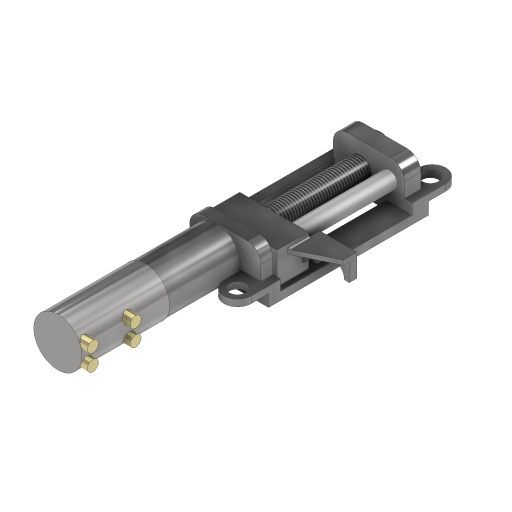
# Autodesk Inventor part: motor_lowest
Saved by Autodesk Inventor 2023 (Build 270158030, 158C)
## iProperties
Created: 2021-04-15
Part Number: motor_lowest
Material: Generic
Document SubType Name: Modeling
Designer: Robert Cobden
Density: 1 g/cm^3
Appearance: Steel Galvanized
Author: Robert Cobden
Autodesk Inventor part; units mm, degrees
sketch "Sketch1" plane through (0, 0, 0) normal (0, 1, 0) x (-1, 0, 0)
  line L0 (3.2, -7.5) -> (-4.7, -7.5)
  line L1 (-4.7, -7.5) -> (-4.7, 7.1)
  line L2 (-4.7, 7.1) -> (3.2, 7.1)
  line L3 (3.2, 7.1) -> (3.2, -7.5)
  line L4 (-2.35, 6) -> (2.35, 6)
  line L5 (2.35, 6) -> (2.35, -6)
  line L6 (2.35, -6) -> (-2.35, -6)
  line L7 (-2.35, -6) -> (-2.35, 6)
  line L8 (-2.35, 6) -> (2.35, -6) construction
  line L9 (2.35, 6) -> (-2.35, -6) construction
  point P0 (0, 0)
  dimension "d0" = 7.9
  dimension "d1" = 14.6
  dimension "d2" = 4.7
  dimension "d3" = 12
  dimension "d4" = 0.85
  dimension "d5" = 1.5
  constraints: 20 end point, 4 parallel, 2 horizontal, 2 midpoint, 2 perpendicular
  measures "d0" distance of L1.end L2.end
  measures "d1" distance of L0.end L1.end
  measures "d2" distance of L5.end L6.end
  measures "d3" distance of L4.end L5.end
  measures "d4" distance between parallel lines of L5 L3
  measures "d5" distance between parallel lines of L0 L6
extrude "Extrusion1" add sketch "Sketch1" along normal blind 0.75
sketch "Sketch2" plane through (0, 0.75, 0) normal (0, 1, 0) x (1, 0, 0)
  line L0 (-3.2, -7.1) -> (4.7, -7.1) projected
  line L1 (4.7, -7.1) -> (4.7, 7.5) projected
  line L2 (4.7, 7.5) -> (-3.2, 7.5) projected
  line L3 (-3.2, 7.5) -> (-3.2, -7.1) projected
  line L4 (2.35, -6) -> (-2.35, -6) projected
  line L5 (-2.35, -6) -> (-2.35, 6) projected
  line L6 (-2.35, 6) -> (2.35, 6) projected
  line L7 (2.35, 6) -> (2.35, -6) projected
  line L8 (-2.35, 6) -> (2.35, 6) projected
  line L9 (2.35, 6) -> (4.7, 6)
  line L10 (4.7, -7.1) -> (4.7, 7.5) projected
  line L11 (2.35, -6) -> (-2.35, -6) projected
  line L12 (2.35, -6) -> (4.7, -6)
  point P0 (0, 0)
  constraints: 4 end point, 2 perpendicular, 2 point on line
extrude "Extrusion2" add sketch "Sketch2" along normal blind 0.95 contours L3 L2 L1 L9 L6 L5 L4 L12 L0
sketch "Sketch3" plane through (0, 1.7, 0) normal (0, 1, 0) x (1, 0, 0)
  line L0 (4.7, -7.1) -> (4.7, -6) projected
  line L1 (4.7, -6) -> (-2.35, -6) projected
  line L2 (-2.35, -6) -> (-2.35, 6) projected
  line L3 (-2.35, 6) -> (4.7, 6) projected
  line L4 (4.7, 6) -> (4.7, 7.5) projected
  line L5 (4.7, 7.5) -> (-3.2, 7.5) projected
  line L6 (-3.2, 7.5) -> (-3.2, -7.1) projected
  line L7 (-3.2, -7.1) -> (4.7, -7.1) projected
  line L8 (4.7, 6) -> (4.7, 7.5) projected
  line L9 (4.7, 7.5) -> (2.2, 7.5)
  line L10 (2.2, 7.5) -> (2.2, 10.34)
  line L11 (2.2, 10.34) -> (4.7, 10.34)
  line L12 (4.7, 10.34) -> (4.7, 7.5)
  line L13 (4.7, 7.5) -> (-3.2, 7.5) projected
  line L14 (-3.2, 7.5) -> (-1.0999, 7.5)
  line L15 (-1.0999, 7.5) -> (-1.0999, 10.2)
  line L16 (-1.0999, 10.2) -> (-3.2, 10.2)
  line L17 (-3.2, 10.2) -> (-3.2, 7.5)
  circle A0 centre (-2.3499, 8.95) radius 1.25
  circle A1 centre (-2.3499, 8.95) radius 0.75
  circle A2 centre (3.45, 8.92) radius 0.75
  line L18 (2.2, 10.34) -> (4.7, 7.5) construction
  line L19 (4.7, -7.1) -> (4.7, 7.5) projected
  line L20 (4.7, -7.1) -> (2.2, -7.1)
  line L21 (2.2, -7.1) -> (2.2, -9.93)
  line L22 (2.2, -9.93) -> (4.7, -9.93)
  line L23 (4.7, -9.93) -> (4.7, -7.1)
  circle A3 centre (3.45, -8.68) radius 0.75
  line L24 (3.45, -9.93) -> (3.45, -8.68) construction
  point P0 (0, 0)
  point P1 (2.2, 7.5)
  point P2 (-3.2, 8.0336)
  point P3 (-1.0999, 7.5)
  point P4 (-2.3499, 10.2)
  dimension "d10" = 2.5
  dimension "d11" = 2.84
  dimension "d12" = 2.1001
  dimension "d13" = 2.7
  dimension "d14" = 2.5
  dimension "d16" = 1.5
  dimension "d17" = 2.5
  dimension "d18" = 2.83
  dimension "d20" = 1.25
  dimension "d38" = 5.8
  dimension "d39" = 8.2999
  dimension "d40" = 7.3
  dimension "d41" = 19.1
  dimension "d42" = 2.17
  dimension "d43" = 2.2
  constraints: 28 end point, 6 parallel, 4 centre point, 3 horizontal, 3 perpendicular, 2 coincident, 2 equal radius, 2 midpoint, 2 tangent, 1 vertical
  measures "d10" distance of L10.end L11.end
  measures "d11" distance of L9.end L10.end
  measures "d12" distance of L16.end L15.end
  measures "d13" distance of L15.end L14.end
  measures "d14" diameter of A0
  measures "d16" diameter of A2
  measures "d17" distance of L22.end L21.end
  measures "d18" distance of L21.end L20.end
  measures "d20" distance of L24.start L24.end
  measures "d38" distance of A2.centre A0.centre
extrude "Extrusion3" add sketch "Sketch3" against normal blind 0.6 contours L23 L22 L21 L7 | L5 L10 L11 L12
extrude "Extrusion4" add sketch "Sketch3" against normal blind 0.4 contours L17 A0 L15 L5 | A0 L17 | L17 A0 | A0 L16 L15
sketch "Sketch4" plane through (0, 1.7, 0) normal (0, 1, 0) x (1, 0, 0)
  circle A0 centre (-2.3499, 8.95) radius 0.75 construction
  circle A1 centre (3.45, -8.68) radius 0.75 construction
  circle A2 centre (3.45, 8.92) radius 0.75 construction
  line L0 (4.7, -9.93) -> (4.7, -6) construction
  line L1 (4.7, -6) -> (-2.35, -6) construction
  line L2 (-2.35, -6) -> (-2.35, 6) construction
  line L3 (-2.35, 6) -> (4.7, 6) construction
  line L4 (4.7, 6) -> (4.7, 10.34) construction
  line L5 (4.7, 10.34) -> (2.2, 10.34) construction
  line L6 (2.2, 10.34) -> (2.2, 7.5) construction
  line L7 (2.2, 7.5) -> (-1.0999, 7.5) construction
  line L8 (-1.0999, 7.5) -> (-1.0999, 10.2) construction
  line L9 (-1.0999, 10.2) -> (-2.3499, 10.2) construction
  arc A3 (-2.3499, 10.2) -> (-3.2, 8.0336) centre (-2.3499, 8.95) ccw construction
  line L10 (-3.2, 8.0336) -> (-3.2, -7.1) construction
  line L11 (-3.2, -7.1) -> (2.2, -7.1) construction
  line L12 (2.2, -7.1) -> (2.2, -9.93) construction
  line L13 (2.2, -9.93) -> (4.7, -9.93) construction
  line L14 (-2.5, 7.5) -> (4, 7.5)
  line L15 (4, 7.5) -> (4, 6)
  line L16 (4, 6) -> (-2.5, 6)
  line L17 (-2.5, 6) -> (-2.5, 7.5)
  line L18 (2.2, 7.5) -> (-1.0999, 7.5) projected
  line L19 (-2.35, 6) -> (4.7, 6) projected
  line L20 (-3.2, 7.5) -> (-3.2, -7.1) construction
  line L21 (-3.2, -1.2421) -> (4.7, -1.2421) construction
  line L22 (-3.2, 8.0336) -> (-3.2, -7.1) construction
  line L23 (4.7, 6) -> (4.7, 10.34) construction
  line L24 (0.75, -1.2421) -> (0.75, 6) construction
  line L25 (-2.5, -6) -> (4, -6)
  line L26 (4, -6) -> (4, -7.1)
  line L27 (4, -7.1) -> (-2.5, -7.1)
  line L28 (-2.5, -7.1) -> (-2.5, -6)
  line L29 (0.75, -1.2421) -> (0.75, -6) construction
  line L30 (4.7, -6) -> (-2.35, -6) construction
  line L31 (-3.2, -7.1) -> (2.2, -7.1) construction
  point P0 (0, 0)
  dimension "d25" = 6.5
  dimension "d26" = 6.5
  constraints: 22 end point, 5 point on line, 4 parallel, 4 perpendicular, 3 midpoint, 2 horizontal, 1 collinear, 1 vertical
  measures "d25" distance of L14.start L14.end
  measures "d26" distance of L26.end L27.end
extrude "Extrusion5" add sketch "Sketch4" along normal blind 2.6
fillet "Fillet1" radius 1.25 5 edges at (2.2, 1.4, 9.93) (4.7, 1.4, 9.93) (4.7, 1.4, -10.34) (2.2, 1.4, -10.34) (-1.0999, 1.5, -10.2)
fillet "Fillet1" radius 1.25 4 edges at (4, 4.3, 6.55) (-2.5, 4.3, 6.55) (-2.5, 4.3, -6.75) (4, 4.3, -6.75)
sketch "Sketch5" plane through (0, 0, 0) normal (0, -1, 0) x (1, 0, 0)
  circle A0 centre (3.55, 5.25) radius 0.55
  circle A1 centre (3.55, -4.8) radius 0.55
  line L0 (4.7, 7.1) -> (4.7, -7.5) projected
  line L1 (3.55, 5.25) -> (3.55, -4.8) construction
  line L2 (4.7, -7.5) -> (-3.2, -7.5) construction
  point P0 (0, 0)
  dimension "d31" = 1.1
  dimension "d33" = 1.7
  dimension "d34" = 11.15
  dimension "d35" = 3.25
  constraints: 2 centre point, 2 end point, 1 equal radius, 1 vertical
  measures "d31" diameter of A1
extrude "Extrusion6" add sketch "Sketch5" along normal blind 0.29
sketch "Sketch6" plane through (-2.35, 0, -6) normal (0, 0, 1) x (1, 0, 0)
  circle A0 centre (4.9823, 2.55) radius 0.75
  circle A1 centre (2.32, 2.15) radius 1
  line L0 (6.35, 1.7) -> (6.35, 3.05) projected
  line L1 (0, 0) -> (4.7, 0) projected
  circle A2 centre (2.32, 2.15) radius 2.15 construction
  line L2 (7.05, 0.75) -> (7.05, 1.7) projected
  line L3 (1.1, 4.3) -> (5.1, 4.3) projected
  point P0 (2.35, 0)
  dimension "d44" = 2.1177
  dimension "d45" = 1.5
  dimension "d46" = 3.3
  dimension "d47" = 2
  dimension "d49" = 4.3
  dimension "d50" = 6.88
  constraints: 3 centre point, 1 coincident, 1 tangent
  measures "d45" diameter of A0
  measures "d47" diameter of A1
  measures "d49" diameter of A2
extrude "Extrusion7" cut sketch "Sketch6" along normal blind 13.1 and the other way blind 1.5 contours A1
extrude "Extrusion8" add sketch "Sketch6" along normal blind 12 contours A0
extrude "Extrusion9" add sketch "Sketch6" along normal blind 13.1 and the other way blind 1.5 separate body contours A1
thread "Thread1" size "M2x0.25" class "6g" standard "ANSI Metric M Profile" full length
sketch "Sketch9" plane through (-3.2, 0, 7.1) normal (0, 0, 1) x (1, 0, 0)
  circle A0 centre (3.17, 2.15) radius 1 construction
  circle A1 centre (3.17, 2.15) radius 2.15
  line L0 (1.95, 4.3) -> (5.95, 4.3) projected
  point P0 (3.2, 0)
  constraints: 1 centre point, 1 coincident, 1 tangent
extrude "Extrusion13" add sketch "Sketch9" along normal blind 6.5 separate body
sketch "Sketch7" plane through (-3.2, 0, 13.6) normal (0, 0, 1) x (1, 0, 0)
  circle A0 centre (3.17, 2.15) radius 1 construction
  circle A1 centre (3.17, 2.15) radius 2.2
  point P0 (3.2, 0)
  dimension "d76" = 4.4
  constraints: 1 centre point, 1 coincident
  measures "d76" diameter of A1
extrude "Extrusion10" add sketch "Sketch7" along normal blind 8 separate body
ref_plane "Work Plane1" through (2.17, 2.15, 13.6) normal (1, 0, 0) x (0, 1, 0)
sketch "Sketch8" plane through (2.17, 2.15, 13.6) normal (1, 0, 0) x (0, 1, 0)
  line L0 (2.2, 8) -> (-2.2, 8) construction
  line L1 (2.2, 0) -> (-2.2, 0) construction
  line L2 (2.2, 0) -> (2.2, 8) construction
  line L3 (-2.2, 0) -> (-2.2, 8) construction
  line L4 (0.75, 7.5) -> (-0.75, 7.5) construction
  line L5 (-0.75, 7.5) -> (-0.75, 3.6) construction
  line L6 (-0.75, 3.6) -> (0.75, 3.6) construction
  line L7 (0.75, 3.6) -> (0.75, 7.5) construction
  line L8 (0.75, 7.5) -> (-0.75, 3.6) construction
  line L9 (0, 5.55) -> (0, 8) construction
  circle A0 centre (0.75, 7.5) radius 0.5
  circle A1 centre (0.75, 3.6) radius 0.5
  circle A2 centre (-0.75, 3.6) radius 0.5
  circle A3 centre (-0.75, 7.5) radius 0.5
  point P0 (-2.15, -13.6)
  dimension "d65" = 3.9
  dimension "d66" = 1.5
  dimension "d67" = 1
  dimension "d68" = 0.5
  constraints: 12 end point, 4 centre point, 4 coincident, 3 equal radius, 2 midpoint, 2 parallel, 2 perpendicular, 1 horizontal
  measures "d65" distance of L6.end L4.start
  measures "d66" distance of L5.end L6.end
  measures "d67" diameter of A1
  measures "d68" distance between parallel lines of L0 L4
extrude "Extrusion11" add sketch "Sketch8" against normal up to surface round surface about axis through (-0.03, 2.15, 13.6) along (0, 0, 1) radius 2.2 far side no bodies 4
extrude "Extrusion12" add sketch "Sketch8" along normal blind 0.5 bodies 4
ref_plane "Work Plane2" through (2.35, 0, 6) normal (0, 0, -1) x (-1, 0, 0)
sketch "Sketch10" plane through (2.35, 0, 6) normal (0, 0, -1) x (-1, 0, 0)
  line L0 (-2.02, 3.8) -> (4.28, 3.8)
  line L1 (4.28, 3.8) -> (4.28, 0)
  line L2 (4.28, 0) -> (-2.02, 0)
  line L3 (-2.02, 0) -> (-2.02, 3.8)
  line L4 (0, 0) -> (4.7, 0) construction
  line L5 (5.55, 0) -> (5.55, 1.7) projected
  line L6 (-2.02, 0) -> (0.48, 0)
  line L7 (0.48, 0) -> (0.48, 0.9)
  line L8 (0.48, 0.9) -> (-2.02, 0.9)
  line L9 (-2.02, 0.9) -> (-2.02, 0)
  circle A0 centre (2.38, 2.15) radius 1 projected
  circle A1 centre (-0.2823, 2.55) radius 0.75 projected
  point P0 (2.35, 0)
  point P1 (-2.02, 0.9)
  dimension "d77" = 6.3
  dimension "d78" = 3.8
  dimension "d81" = 3.8
  dimension "d82" = 2.9
  dimension "d83" = 1.9
  constraints: 16 end point, 4 parallel, 2 horizontal, 2 perpendicular, 1 point on line
  measures "d77" distance of L1.end L2.end
  measures "d78" distance of L0.end L1.end
  measures "d81" distance between parallel lines of L1 L7
  measures "d82" distance between parallel lines of L0 L8
  measures "d83" distance from line of L1 A0.centre
extrude "Extrusion14" add sketch "Sketch10" along normal blind 2.9 separate body contours L0 L1 L2 L7 L8 L3
thread "Thread2" size "M2x0.4" class "6H" standard "ANSI Metric M Profile" full length
ref_plane "Work Plane3" through (-1.93, 3.4, 6) normal (0, 1, 0) x (1, 0, 0)
sketch "Sketch11" plane through (-1.93, 3.4, 6) normal (0, 1, 0) x (1, 0, 0)
  line L0 (6.3, 0) -> (6.3, 2.9) construction
  line L1 (6.3, 0) -> (6.3, 2.9) construction
  line L2 (6.3, 3.9) -> (9.7, 3.9)
  line L3 (9.7, 3.9) -> (9.7, 1)
  line L4 (9.7, 1) -> (6.3, 1)
  line L5 (6.3, 1) -> (6.3, 3.9)
  line L6 (6.3, 1) -> (9.7, 2.65)
  point P0 (1.93, 6)
  dimension "d89" = 3.4
  dimension "d90" = 2.9
  dimension "d91" = 3.9
  dimension "d92" = 1.25
  constraints: 10 end point, 2 parallel, 2 point on line, 1 horizontal, 1 perpendicular
  measures "d89" distance of L3.end L4.end
  measures "d90" distance of L2.end L3.end
  measures "d91" distance from line of L2 L1.start
  measures "d92" distance of L2.end L6.end
extrude "Extrusion15" add sketch "Sketch11" against normal blind 0.4 contours L2 L3 L6 L5 bodies 5
sketch "Sketch12" plane through (7.77, 3.4, 2.1) normal (0, 0, -1) x (-1, 0, 0)
  line L0 (0, 0) -> (3.4, 0) construction
  line L1 (0, 0) -> (0, -0.4) construction
  line L2 (3.4, -0.4) -> (0, -0.4) construction
  line L3 (3.4, 0) -> (3.4, -0.4) construction
  line L4 (0, -0.4) -> (3.4, -0.4)
  line L5 (3.4, -0.4) -> (3.4, -2.05)
  line L6 (3.4, -2.05) -> (0, -2.05)
  line L7 (0, -2.05) -> (0, -0.4)
  circle A0 centre (1.7, -2.05) radius 1.25
  point P0 (7.77, -3.4)
  point P1 (0.45, -2.05)
  point P2 (2.95, -2.05)
  dimension "d95" = 2.5
  dimension "d96" = 0.4
  constraints: 8 end point, 2 parallel, 1 centre point, 1 horizontal, 1 midpoint, 1 perpendicular, 1 point on line
  measures "d95" diameter of A0
  measures "d96" distance edge to line of A0 L4
extrude "Extrusion16" add sketch "Sketch12" against normal blind 0.7 contours L4 L5 L6 A0 L7 bodies 5
sketch "Sketch13" plane through (7.77, 3.4, 2.8) normal (0, 0, 1) x (1, 0, 0)
  line L0 (-3.4, -0.4) -> (-1.4, -0.4)
  line L1 (-1.4, -0.4) -> (-1.4, -1.7)
  line L2 (-1.4, -1.7) -> (-3.4, -1.7)
  line L3 (-3.4, -1.7) -> (-3.4, -0.4)
  circle A0 centre (-1.7, -2.05) radius 1.4166
  line L4 (-3.4, -0.4) -> (0, -0.4) construction
  line L5 (-3.4, -0.4) -> (-3.4, -2.05) construction
  line L6 (-3.4, -2.05) -> (-2.95, -2.05) construction
  arc A1 (-0.45, -2.05) -> (-2.95, -2.05) centre (-1.7, -2.05) ccw construction
  line L7 (-0.45, -2.05) -> (0, -2.05) construction
  line L8 (0, -2.05) -> (0, -0.4) construction
  point P0 (-7.77, -3.4)
  point P1 (-3.0726, -1.7)
  point P2 (-1.4, -0.6656)
  dimension "d99" = 2
  dimension "d100" = 1.3
  constraints: 8 end point, 2 parallel, 1 centre point, 1 coincident, 1 horizontal, 1 perpendicular
  measures "d99" distance of L1.end L2.end
  measures "d100" distance of L0.end L1.end
extrude "Extrusion17" add sketch "Sketch13" along normal blind 0.9 contours L0 L1 A0 L2 L3 bodies 5
fillet "Fillet2" radius 1.25 2 edges at (6.37, 2.7344, 3.25) (4.6974, 1.7, 3.25)
fillet "Fillet2" radius 0.25 1 edges at (4.37, 3.4, 4.05)
sketch "Sketch15" plane through (7.77, 3.4, 2.1) normal (0, 0, -1) x (-1, 0, 0)
  line L0 (0, 0) -> (3.4, 0) projected
  line L1 (0, 0) -> (0, -2.05) projected
  line L2 (0, -2.05) -> (0.45, -2.05) projected
  arc A0 (2.95, -2.05) -> (0.45, -2.05) centre (1.7, -2.05) ccw projected
  line L3 (2.95, -2.05) -> (3.4, -2.05) projected
  line L4 (3.4, 0) -> (3.4, -2.05) projected
  circle A1 centre (1.7, -2.05) radius 1.25
  point P0 (7.77, -3.4)
  constraints: 1 centre point, 1 coincident
equation "\"CPos\" = 0"
body "Solid1"
body "Solid2"
body "Solid3"
body "Solid6"
body "Solid7"
